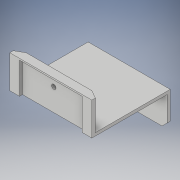
# Autodesk Inventor part: battery-strap casing
Saved by Autodesk Inventor 2019 (Build 230136000, 136)
## iProperties
Created: 2020-04-12
Part Number: battery-strap casing
Material: Generic
Document SubType Name: Modeling
Designer: Jorge
Density: 1 g/cm^3
Appearance: Default
Author: Jorge
Autodesk Inventor part; units mm, degrees
ref_plane "YZ Plane" through (0, 0, 0) normal (1, 0, 0) x (0, 1, 0)
ref_plane "XZ Plane" through (0, 0, 0) normal (0, 1, 0) x (-1, 0, 0)
ref_plane "XY Plane" through (0, 0, 0) normal (0, 0, 1) x (1, 0, 0)
sketch "Sketch1" plane through (0, 0, 0) normal (0, 0, 1) x (1, 0, 0)
  circle A0 centre (0, 0) radius 1.5
  line L0 (-22, 7) -> (22, 7)
  line L1 (0, -11.4299) -> (0, 7) construction
  line L2 (-22, 7) -> (-22, -13)
  line L3 (-44.6409, -15) -> (38.9011, -15) construction
  line L4 (22, 7) -> (22, -13)
  line L5 (-22, -13) -> (-21, -13)
  line L6 (-21, -13) -> (-21, 6)
  line L7 (-21, 6) -> (21, 6)
  line L8 (21, 6) -> (21, -13)
  line L9 (21, -13) -> (22, -13)
  line L10 (-21, -13) -> (21, -13)
  line L11 (-27.5, -15) -> (27.5, -15)
  line L12 (-27.5, -15) -> (-27.5, -13)
  line L13 (-27.5, -13) -> (-21, -13)
  line L14 (22, -13) -> (27.5, -13)
  line L15 (27.5, -13) -> (27.5, -15)
  point P0 (0, -15)
  dimension "d0" = 3
  dimension "d1" = 7
  dimension "d2" = 44
  dimension "d3" = 20
  dimension "d4" = 15
  dimension "d5" = 1
  dimension "d8" = 1
  dimension "d9" = 1
  dimension "d10" = 55
  constraints: 32 end point, 6 perpendicular, 6 point on line, 4 horizontal, 4 vertical, 2 midpoint, 1 centre point, 1 coincident, 1 parallel
  measures "d0" diameter of A0
  measures "d1" distance from line of L0 point (0, 0)
  measures "d2" distance of L0.start L0.end
  measures "d3" distance of L0.start L2.end
  measures "d4" distance from line of L3 point (0, 0)
  measures "d5" distance of L2.end L5.end
  measures "d8" distance between parallel lines of L0 L7
  measures "d9" distance between parallel lines of L4 L8
  measures "d10" distance of L11.start L11.end
extrude "Extrusion1" add sketch "Sketch1" along normal blind 5.5 contours L0 L4 L9 L8 L7 L6 L5 L2
extrude "Extrusion2" add sketch "Sketch1" along normal blind 3.5 contours L6 L7 L8 L10
extrude "Extrusion3" add sketch "Sketch1" along normal blind 3.5 and the other way blind 47 contours L5 L10 L9 L14 L15 L11 L12 L13
draft "FaceDraft1" angle 60 pull direction (0, 0, -1) fixed plane through (-0.0603, -9.163, 0) normal (0, 0, -1) faces at (22, 0.3333, 3) (-22, 0.3333, 3)
sketch "Sketch2" plane through (-27.5, -15, 3.5) normal (0, -1, 0) x (1, 0, 0)
  line L0 (55, -50.5) -> (55, 0) construction
  line L1 (0, 0) -> (55, 0) construction
  line L2 (0, -50.5) -> (0, 0) construction
  line L3 (55, -50.5) -> (0, -50.5) construction
  line L4 (0, -50.5) -> (55, -50.5) projected
  line L5 (0, -50.5) -> (0, 0) projected
  line L6 (55, -50.5) -> (0, -50.5)
  line L7 (0, -50.5) -> (0, -48.5)
  line L8 (0, -48.5) -> (55, -48.5)
  line L9 (55, -48.5) -> (55, -50.5)
  point P0 (27.5, -3.5)
  dimension "d20" = 2
  constraints: 8 end point, 2 parallel, 1 horizontal, 1 perpendicular, 1 point on line
  measures "d20" distance of L6.end L7.end
extrude "Extrusion4" add sketch "Sketch2" along normal blind 20
move faces "Move1" translate (0, -2, 0) faces at (26.6754, -13, 4.8333) (-26.6754, -13, 4.8333)
ref_plane "Work Plane1" through (27.5, -15, -47) normal (1, 0, 0) x (0, -1, 0)
ref_plane "Work Plane2" through (-27.5, -15, -45) normal (-1, 0, 0) x (0, -1, 0)
split "Split1" plane through (27.5, -15, -47) removes the side toward (1, 0, 0)
split "Split2" plane through (-27.5, -15, -45) removes the side toward (-1, 0, 0)
chamfer "Chamfer1" distance 3.5 angle 45 2 edges at (-27.5, -35, -46) (27.5, -35, -46)
body "Solid1"
